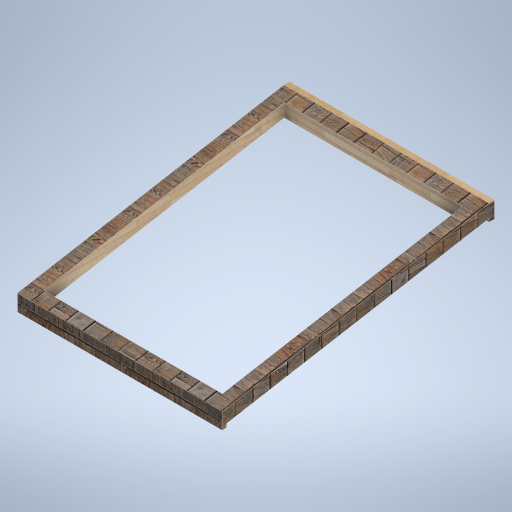
# Autodesk Inventor part: eave_frame_02
Saved by Autodesk Inventor 2024.3 (Build 283343000, 343)
## iProperties
Created: 2024-05-23
Part Number: eave_frame_02
Material: Wood (Maple)
Document SubType Name: Modeling
Designer: Huang
Density: 0.67 g/cm^3
Appearance: Natural Maple - Glossy Dark Tint
Author: Huang
Autodesk Inventor part; units mm, degrees
ref_plane "YZ Plane" through (0, 0, 0) normal (1, 0, 0) x (0, 1, 0)
ref_plane "XZ Plane" through (0, 0, 0) normal (0, 1, 0) x (-1, 0, 0)
sketch "Sketch2" plane through (0, 0, 0) normal (0, 0, 1) x (1, 0, 0)
  line L0 (-4731.265, 1505.8501) -> (4722.9578, 1505.8501)
  line L1 (2684.4021, 1074.0253) -> (2684.4021, 1505.8501)
  line L2 (4412.9578, -1494.1499) -> (4412.9578, 1505.8501)
  line L3 (4722.9578, -1494.1499) -> (4722.9578, 1505.8501)
  line L4 (4412.9578, 1505.8501) -> (4722.9578, 1505.8501)
  line L5 (4567.9578, 1505.8501) -> (4567.9578, 1355.8501)
  line L6 (4567.9578, 1355.8501) -> (2684.4021, 1355.8501)
  point P0 (0, 0)
  dimension "d0" = 150
  constraints: 14 end point, 1 coincident, 1 collinear, 1 midpoint, 1 perpendicular, 1 point on line, 1 vertical
  measures "d0" distance of L5.start L5.end
ref_plane "Work Plane2" through (0, 0, 2500) normal (0, 0, 1) x (1, 0, 0)
ref_plane "Work Plane1" through (0, 0, 0) normal (0, 0, 1) x (1, 0, 0)
sketch "Sketch3" plane through (0, 0, 2500) normal (0, 0, 1) x (1, 0, 0)
  line L0 (2684.4021, 1074.0253) -> (2684.4021, 1505.8501) projected
  point P0 (0, 0)
extrude "Extrusion1" add sketch "Sketch2" along normal blind 51
ref_plane "Work Plane3" through (4722.9578, 1505.8501, 51) normal (0, 0, 1) x (-1, 0, 0)
sketch "Sketch4" plane through (4722.9578, 1505.8501, 51) normal (0, 0, 1) x (-1, 0, 0)
  line L0 (155, 150) -> (155, 0) projected
  line L1 (155, 0) -> (2038.5557, 0) projected
  line L2 (2038.5557, 0) -> (2038.5557, 150) projected
  line L3 (2038.5557, 150) -> (155, 150) projected
  line L4 (2038.5557, 150) -> (155, 150) projected
  line L5 (2038.5557, 0) -> (155, 0)
  line L6 (155, 0) -> (155, 150)
  line L7 (155, 150) -> (2038.5557, 150)
  line L8 (2038.5557, 150) -> (2038.5557, 0)
  point P0 (4722.9578, 1505.8501)
  constraints: 8 end point, 2 parallel, 1 horizontal, 1 perpendicular
ref_plane "Work Plane4" through (2684.4021, 1505.8501, 51) normal (-1, 0, 0) x (0, -1, 0)
sketch "Sketch5" plane through (2684.4021, 1505.8501, 51) normal (-1, 0, 0) x (0, -1, 0)
  line L0 (150, 0) -> (0, 0) projected
  line L1 (0, 0) -> (150, 0) projected
  line L2 (0, 0) -> (150, 0)
  line L3 (431.8248, 2449) -> (0, 2449) projected
  line L4 (431.8248, 2449) -> (581.8248, 2449)
  line L5 (0, 0) -> (431.8248, 2449)
  line L6 (0, 0) -> (2486.7798, 0) construction
  line L7 (150, 0) -> (581.8248, 2449)
  line L8 (150, 0) -> (2636.7798, 0) construction
  point P0 (1505.8501, -51)
  dimension "d5" = 80
  dimension "d6" = 80
  constraints: 12 end point, 3 horizontal, 2 coincident, 2 equal length, 1 collinear
  measures "d5" angle of L6 L5
  measures "d6" angle of L8 L7
sketch "Sketch6" plane through (0, 0, 2500) normal (0, 0, 1) x (1, 0, 0)
  line L0 (2684.4021, 1074.0253) -> (2684.4021, 924.0253) projected
  line L1 (4567.9578, 1074.0253) -> (4567.9578, 924.0253)
  line L2 (2684.4021, 1074.0253) -> (4567.9578, 1074.0253)
  line L3 (2684.4021, 924.0253) -> (4567.9578, 924.0253)
  line L4 (4567.9578, 1074.0253) -> (4567.9578, 924.0253)
  line L5 (2684.4021, 1074.0253) -> (4567.9578, 1074.0253)
  line L6 (4567.9578, 1074.0253) -> (4567.9578, 924.0253)
  line L7 (4567.9578, 924.0253) -> (2684.4021, 924.0253)
  line L8 (2684.4021, 924.0253) -> (2684.4021, 1074.0253)
  point P0 (0, 0)
  constraints: 16 end point, 3 perpendicular, 2 coincident, 2 parallel, 1 horizontal, 1 vertical
loft "Loft1" add profiles "Sketch6" section 2 edges at (4567.9578, 1430.8501, 51) (3626.18, 1505.8501, 51) (2684.4021, 1430.8501, 51) (3626.18, 1355.8501, 51)
sketch "Sketch7" plane through (2684.4021, 1505.8501, 51) normal (-1, 0, 0) x (0, -1, 0)
  line L0 (0, 0) -> (150, 0) projected
  line L1 (581.8248, 2449) -> (150, 0) projected
  line L2 (431.8248, 2449) -> (581.8248, 2449) projected
  line L3 (499.9267, 2449) -> (499.9267, 2413)
  line L4 (545.477, 2413) -> (575.477, 2413)
  line L5 (150, 0) -> (120, 0)
  line L6 (120, 0) -> (545.477, 2413)
  line L7 (120, 0) -> (2570.2244, 0) construction
  line L8 (150, 0) -> (575.477, 2413)
  line L9 (545.477, 2413) -> (575.477, 2413)
  line L10 (545.477, 2413) -> (575.477, 2413)
  line L11 (150, -51) -> (0, -51) projected
  point P0 (1505.8501, -51)
  dimension "d11" = 36
  dimension "d12" = 30
  dimension "d13" = 80
  constraints: 16 end point, 3 point on line, 1 coincident, 1 collinear, 1 equal length, 1 horizontal, 1 parallel, 1 perpendicular, 1 vertical
  measures "d11" distance of L3.start L3.end
  measures "d12" distance of L0.end L5.end
  measures "d13" angle of L7 L6
extrude "Extrusion2" cut sketch "Sketch7" against normal through all
ref_plane "Work Plane5" through (4722.9578, 1505.8501, 0) normal (0, 1, 0) x (-1, 0, 0)
sketch "Sketch8" plane through (4722.9578, 1505.8501, 0) normal (0, 1, 0) x (-1, 0, 0)
  line L0 (155, 2500) -> (2038.5557, 2500) projected
  line L1 (155, 2500) -> (155, 51) projected
  line L2 (155, 51) -> (2038.5557, 51) projected
  line L3 (2038.5557, 2500) -> (2038.5557, 51) projected
  line L4 (2038.5557, 51) -> (2038.5557, 2464) projected
  line L5 (2038.5557, 51) -> (1918.5557, 51)
  line L6 (1918.5557, 51) -> (1918.5557, 171)
  line L7 (1918.5557, 171) -> (2038.5557, 171)
  line L8 (2038.5557, 171) -> (2038.5557, 51)
  line L9 (155, 2500) -> (275, 2500)
  line L10 (275, 2500) -> (275, 2380)
  line L11 (275, 2380) -> (155, 2380)
  line L12 (155, 2380) -> (155, 2500)
  line L13 (1918.5557, 171) -> (275, 171)
  line L14 (275, 171) -> (275, 2380)
  line L15 (275, 2380) -> (1918.5557, 2380)
  line L16 (1918.5557, 2380) -> (1918.5557, 171)
  point P0 (4722.9578, 0)
  dimension "d16" = 120
  dimension "d17" = 120
  dimension "d18" = 120
  dimension "d19" = 120
  constraints: 24 end point, 6 parallel, 3 horizontal, 3 perpendicular
  measures "d16" distance of L6.end L7.end
  measures "d17" distance of L5.end L6.end
  measures "d18" distance of L10.end L11.end
  measures "d19" distance of L9.end L10.end
extrude "Extrusion3" cut sketch "Sketch8" against normal through all contours L15 L16 L13 L14
body "Solid1"
